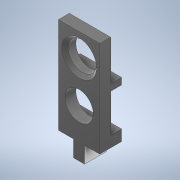
# Autodesk Inventor part: LED-Spacer1
Saved by Autodesk Inventor 2022 (Build 260153000, 153)
## iProperties
Created: 2024-06-27
Part Number: LED-Spacer1
Material: 一般
Document SubType Name: Modeling
Designer: yamashita1
Density: 1 g/cm^3
Appearance: 既定
Author: yamashita1
Autodesk Inventor part; units mm, degrees
ref_plane "YZ Plane" through (0, 0, 0) normal (1, 0, 0) x (0, 1, 0)
ref_plane "XZ Plane" through (0, 0, 0) normal (0, 1, 0) x (-1, 0, 0)
ref_plane "XY Plane" through (0, 0, 0) normal (0, 0, 1) x (1, 0, 0)
sketch "スケッチ1" plane through (0, 0, 0) normal (0, 0, 1) x (1, 0, 0)
  circle A0 centre (0, 5.8) radius 2.6
  circle A1 centre (0, 13.4) radius 2.6
  line L0 (-3.8, 0) -> (3.8, 0)
  line L1 (3.8, 0) -> (3.8, 17.6)
  line L2 (3.8, 17.6) -> (-3.8, 17.6)
  line L3 (-3.8, 17.6) -> (-3.8, 0)
  line L4 (-11.5586, 9.6) -> (11.5586, 9.6) construction
  point P0 (0, 0)
  point P1 (0, 0)
  point P2 (0, 9.6)
  dimension "LED_DIA" = 5.2
  dimension "d1" = 7.6
  dimension "LED_PITCH" = 7.6
  dimension "TOP_MARGIN" = 4.2
  dimension "BOTTOM_MARGIN" = 5.8
  constraints: 10 end point, 2 centre point, 2 horizontal, 2 midpoint, 2 parallel, 2 vertical alignment, 1 coincident, 1 equal radius, 1 perpendicular, 1 symmetric about line
  measures "LED_DIA" diameter of A0
  measures "d1" distance of L0.start L0.end
  measures "LED_PITCH" distance of A1.centre A0.centre
  measures "TOP_MARGIN" distance from line of L2 A1.centre
  measures "BOTTOM_MARGIN" distance from line of L0 A0.centre
extrude "スペーサ" add sketch "スケッチ1" along normal blind 2
sketch "スケッチ2" plane through (0, 0, 0) normal (0, 0, -1) x (-1, 0, 0)
  line L0 (3.8, 17.6) -> (3.8, 0) projected
  line L1 (-3.8, 0) -> (-3.8, 17.6) projected
  line L2 (3.8, 0) -> (-3.8, 0)
  line L3 (-3.8, 0) -> (-3.8, 2)
  line L4 (-3.8, 2) -> (3.8, 2)
  line L5 (3.8, 2) -> (3.8, 0)
  line L6 (3.8, 10.2) -> (-3.8, 10.2)
  line L7 (-3.8, 10.2) -> (-3.8, 9)
  line L8 (-3.8, 9) -> (3.8, 9)
  line L9 (3.8, 9) -> (3.8, 10.2)
  circle A0 centre (0, 5.8) radius 2.9 construction
  circle A1 centre (0, 13.4) radius 2.9 construction
  circle A2 centre (0, 5.8) radius 2.6 construction
  circle A3 centre (0, 13.4) radius 2.6 construction
  line L10 (6.2058, 13.4) -> (-6.2058, 13.4) construction
  line L11 (-6.2058, 5.8) -> (6.2058, 5.8) construction
  line L12 (6.2058, 9.6) -> (-6.2058, 9.6) construction
  point P0 (0, 0)
  point P1 (3.8, 9.6)
  point P2 (-3.8, 9)
  point P3 (3.8, 9)
  point P4 (3.8, 10.2)
  point P5 (-3.8, 10.2)
  dimension "d8" = 5.8
  dimension "d9" = 2
  dimension "d10" = 1.2
  constraints: 22 end point, 5 horizontal, 4 parallel, 4 point on line, 3 midpoint, 2 centre point, 2 coincident, 2 concentric, 2 perpendicular, 1 equal radius, 1 other
  measures "d8" diameter of A0
  measures "d9" distance between parallel lines of L2 L4
  measures "d10" distance of L6.end L7.end
extrude "押し出し2" add sketch "スケッチ2" along normal blind 2 contours L0 L8 L1 L6 | L0 L2 L1 L4
chamfer "面取り1" distance 0.6 angle 45 1 edges at (-2.6, 13.4, 2)
sketch "スケッチ3" plane through (-3.8, 0, 2) normal (0, -1, 0) x (1, 0, 0)
  line L0 (0, 0) -> (7.6, 0) projected
  line L1 (7.6, -4) -> (0, -4) projected
  line L2 (4.8, 0) -> (2.8, 0)
  line L3 (2.8, 0) -> (2.8, -4)
  line L4 (2.8, -4) -> (4.8, -4)
  line L5 (4.8, -4) -> (4.8, 0)
  point P0 (3.8, -2)
  point P1 (3.8, 0)
  dimension "d16" = 2
  constraints: 8 end point, 2 parallel, 2 point on line, 1 horizontal, 1 midpoint, 1 perpendicular, 1 vertical alignment
  measures "d16" distance between parallel lines of L3 L5
extrude "押し出し3" add sketch "スケッチ3" along normal blind 3
